Autodesk Fusion 360 part; units mm, degrees
(part 3 of 3)
sketch "b left circles" plane through (0, 0, 0) normal (0, 0, 1) x (1, 0, 0) in component "b left component"
  line L0 (104.02, 122.01) -> (154.02, 122.01)
  line L1 (154.02, 122.01) -> (154.02, 242.01)
  line L2 (154.02, 242.01) -> (104.02, 242.01)
  line L3 (104.02, 242.01) -> (104.02, 122.01)
  circle A0 centre (114.7106, 124.3744) radius 1.005
  circle A1 centre (123.3294, 124.3744) radius 1.005
  circle A2 centre (134.7106, 124.3744) radius 1.005
  circle A3 centre (143.3294, 124.3744) radius 1.005
  circle A4 centre (151.6556, 136.3194) radius 1.005
  circle A5 centre (151.6556, 147.7006) radius 1.005
  circle A6 centre (151.6556, 156.3194) radius 1.005
  circle A7 centre (151.6556, 167.7006) radius 1.005
  circle A8 centre (151.6556, 176.3194) radius 1.005
  circle A9 centre (151.6556, 187.7006) radius 1.005
  circle A10 centre (151.6556, 196.3194) radius 1.005
  circle A11 centre (151.6556, 207.7006) radius 1.005
  circle A12 centre (151.6556, 216.3194) radius 1.005
  circle A13 centre (151.6556, 227.7006) radius 1.005
  circle A14 centre (114.7106, 239.6456) radius 1.005
  circle A15 centre (123.3294, 239.6456) radius 1.005
  circle A16 centre (134.7106, 239.6456) radius 1.005
  circle A17 centre (143.3294, 239.6456) radius 1.005
  circle A18 centre (106.3844, 136.3194) radius 1.005
  circle A19 centre (106.3844, 147.7006) radius 1.005
  circle A20 centre (106.3844, 156.3194) radius 1.005
  circle A21 centre (106.3844, 167.7006) radius 1.005
  circle A22 centre (106.3844, 176.3194) radius 1.005
  circle A23 centre (106.3844, 187.7006) radius 1.005
  circle A24 centre (106.3844, 196.3194) radius 1.005
  circle A25 centre (106.3844, 207.7006) radius 1.005
  circle A26 centre (106.3844, 216.3194) radius 1.005
  circle A27 centre (106.3844, 227.7006) radius 1.005
  dimension "d1976" = 2.01
  dimension "d1977" = 2.01
  dimension "d1978" = 2.01
  dimension "d1979" = 2.01
  dimension "d2001" = 2.01
  dimension "d2002" = 2.01
  dimension "d2003" = 2.01
  dimension "d2004" = 2.01
  dimension "d2005" = 2.01
  dimension "d2006" = 2.01
  dimension "d2007" = 2.01
  dimension "d2008" = 2.01
  dimension "d2009" = 2.01
  dimension "d2010" = 2.01
  dimension "d2020" = 2.01
  dimension "d2021" = 2.01
  dimension "d2022" = 2.01
  dimension "d2023" = 2.01
  dimension "d2045" = 2.01
  dimension "d2046" = 2.01
  dimension "d2047" = 2.01
  dimension "d2048" = 2.01
  dimension "d2049" = 2.01
  dimension "d2050" = 2.01
  dimension "d2051" = 2.01
  dimension "d2052" = 2.01
  dimension "d2053" = 2.01
  dimension "d2054" = 2.01
  measures "d1976" diameter of A0
  measures "d1977" diameter of A1
  measures "d1978" diameter of A2
  measures "d1979" diameter of A3
  measures "d2001" diameter of A4
  measures "d2002" diameter of A5
  measures "d2003" diameter of A6
  measures "d2004" diameter of A7
  measures "d2005" diameter of A8
  measures "d2006" diameter of A9
  measures "d2007" diameter of A10
  measures "d2008" diameter of A11
  measures "d2009" diameter of A12
  measures "d2010" diameter of A13
  measures "d2020" diameter of A14
  measures "d2021" diameter of A15
  measures "d2022" diameter of A16
  measures "d2023" diameter of A17
  measures "d2045" diameter of A18
  measures "d2046" diameter of A19
  measures "d2047" diameter of A20
  measures "d2048" diameter of A21
  measures "d2049" diameter of A22
  measures "d2050" diameter of A23
  measures "d2051" diameter of A24
  measures "d2052" diameter of A25
  measures "d2053" diameter of A26
  measures "d2054" diameter of A27
extrude "b left lines body extrude" add sketch "b left lines" along normal blind 3.175 separate body makes body 10 in component "b left component"
extrude "b left circles extrude" add sketch "b left circles" along normal blind 3.175 separate body makes body 11 in component "b left component"
combine "b left lines final combine feature" operation intersect target body 10 tool bodies 11 in component "b left component"
sketch "b right lines" plane through (0, 0, 0) normal (0, 0, 1) x (1, 0, 0) in component "b right component"
  line L0 (159.205, 122.01) -> (166.13, 122.01)
  line L1 (166.13, 122.01) -> (166.13, 125.185)
  line L2 (166.13, 125.185) -> (175.93, 125.185)
  line L3 (175.93, 125.185) -> (175.93, 122.01)
  line L4 (175.93, 122.01) -> (186.13, 122.01)
  line L5 (186.13, 122.01) -> (186.13, 125.185)
  line L6 (186.13, 125.185) -> (195.93, 125.185)
  line L7 (195.93, 125.185) -> (195.93, 122.01)
  line L8 (195.93, 122.01) -> (202.855, 122.01)
  line L9 (202.855, 122.01) -> (202.855, 136.91)
  line L10 (202.855, 136.91) -> (206.03, 136.91)
  line L11 (206.03, 136.91) -> (206.03, 147.11)
  line L12 (206.03, 147.11) -> (202.855, 147.11)
  line L13 (202.855, 147.11) -> (202.855, 156.91)
  line L14 (202.855, 156.91) -> (206.03, 156.91)
  line L15 (206.03, 156.91) -> (206.03, 167.11)
  line L16 (206.03, 167.11) -> (202.855, 167.11)
  line L17 (202.855, 167.11) -> (202.855, 176.91)
  line L18 (202.855, 176.91) -> (206.03, 176.91)
  line L19 (206.03, 176.91) -> (206.03, 187.11)
  line L20 (206.03, 187.11) -> (202.855, 187.11)
  line L21 (202.855, 187.11) -> (202.855, 196.91)
  line L22 (202.855, 196.91) -> (206.03, 196.91)
  line L23 (206.03, 196.91) -> (206.03, 207.11)
  line L24 (206.03, 207.11) -> (202.855, 207.11)
  line L25 (202.855, 207.11) -> (202.855, 216.91)
  line L26 (202.855, 216.91) -> (206.03, 216.91)
  line L27 (206.03, 216.91) -> (206.03, 227.11)
  line L28 (206.03, 227.11) -> (202.855, 227.11)
  line L29 (202.855, 227.11) -> (202.855, 242.01)
  line L30 (159.205, 242.01) -> (166.13, 242.01)
  line L31 (166.13, 242.01) -> (166.13, 238.835)
  line L32 (166.13, 238.835) -> (175.93, 238.835)
  line L33 (175.93, 238.835) -> (175.93, 242.01)
  line L34 (175.93, 242.01) -> (186.13, 242.01)
  line L35 (186.13, 242.01) -> (186.13, 238.835)
  line L36 (186.13, 238.835) -> (195.93, 238.835)
  line L37 (195.93, 238.835) -> (195.93, 242.01)
  line L38 (195.93, 242.01) -> (202.855, 242.01)
  line L39 (159.205, 122.01) -> (159.205, 136.91)
  line L40 (159.205, 136.91) -> (156.03, 136.91)
  line L41 (156.03, 136.91) -> (156.03, 147.11)
  line L42 (156.03, 147.11) -> (159.205, 147.11)
  line L43 (159.205, 147.11) -> (159.205, 156.91)
  line L44 (159.205, 156.91) -> (156.03, 156.91)
  line L45 (156.03, 156.91) -> (156.03, 167.11)
  line L46 (156.03, 167.11) -> (159.205, 167.11)
  line L47 (159.205, 167.11) -> (159.205, 176.91)
  line L48 (159.205, 176.91) -> (156.03, 176.91)
  line L49 (156.03, 176.91) -> (156.03, 187.11)
  line L50 (156.03, 187.11) -> (159.205, 187.11)
  line L51 (159.205, 187.11) -> (159.205, 196.91)
  line L52 (159.205, 196.91) -> (156.03, 196.91)
  line L53 (156.03, 196.91) -> (156.03, 207.11)
  line L54 (156.03, 207.11) -> (159.205, 207.11)
  line L55 (159.205, 207.11) -> (159.205, 216.91)
  line L56 (159.205, 216.91) -> (156.03, 216.91)
  line L57 (156.03, 216.91) -> (156.03, 227.11)
  line L58 (156.03, 227.11) -> (159.205, 227.11)
  line L59 (159.205, 227.11) -> (159.205, 242.01)
  dimension "d2059" = 6.925
  dimension "d2060" = 3.175
  dimension "d2061" = 9.8
  dimension "d2062" = 3.175
  dimension "d2063" = 10.2
  dimension "d2064" = 3.175
  dimension "d2065" = 9.8
  dimension "d2066" = 3.175
  dimension "d2067" = 6.925
  dimension "d2072" = 14.9
  dimension "d2073" = 3.175
  dimension "d2074" = 10.2
  dimension "d2075" = 3.175
  dimension "d2076" = 9.8
  dimension "d2077" = 3.175
  dimension "d2078" = 10.2
  dimension "d2079" = 3.175
  dimension "d2080" = 9.8
  dimension "d2081" = 3.175
  dimension "d2082" = 10.2
  dimension "d2083" = 3.175
  dimension "d2084" = 9.8
  dimension "d2085" = 3.175
  dimension "d2086" = 10.2
  dimension "d2087" = 3.175
  dimension "d2088" = 9.8
  dimension "d2089" = 3.175
  dimension "d2090" = 10.2
  dimension "d2091" = 3.175
  dimension "d2092" = 14.9
  dimension "d2103" = 6.925
  dimension "d2104" = 3.175
  dimension "d2105" = 9.8
  dimension "d2106" = 3.175
  dimension "d2107" = 10.2
  dimension "d2108" = 3.175
  dimension "d2109" = 9.8
  dimension "d2110" = 3.175
  dimension "d2111" = 6.925
  dimension "d2116" = 14.9
  dimension "d2117" = 3.175
  dimension "d2118" = 10.2
  dimension "d2119" = 3.175
  dimension "d2120" = 9.8
  dimension "d2121" = 3.175
  dimension "d2122" = 10.2
  dimension "d2123" = 3.175
  dimension "d2124" = 9.8
  dimension "d2125" = 3.175
  dimension "d2126" = 10.2
  dimension "d2127" = 3.175
  dimension "d2128" = 9.8
  dimension "d2129" = 3.175
  dimension "d2130" = 10.2
  dimension "d2131" = 3.175
  dimension "d2132" = 9.8
  dimension "d2133" = 3.175
  dimension "d2134" = 10.2
  dimension "d2135" = 3.175
  dimension "d2136" = 14.9
  constraint horizontal L0
  constraint vertical L1
  constraint horizontal L2
  constraint vertical L3
  constraint horizontal L4
  constraint vertical L5
  constraint horizontal L6
  constraint vertical L7
  constraint horizontal L8
  constraint vertical L9
  constraint horizontal L10
  constraint vertical L11
  constraint horizontal L12
  constraint vertical L13
  constraint horizontal L14
  constraint vertical L15
  constraint horizontal L16
  constraint vertical L17
  constraint horizontal L18
  constraint vertical L19
  constraint horizontal L20
  constraint vertical L21
  constraint horizontal L22
  constraint vertical L23
  constraint horizontal L24
  constraint vertical L25
  constraint horizontal L26
  constraint vertical L27
  constraint horizontal L28
  constraint vertical L29
  constraint horizontal L30
  constraint vertical L31
  constraint horizontal L32
  constraint vertical L33
  constraint horizontal L34
  constraint vertical L35
  constraint horizontal L36
  constraint vertical L37
  constraint horizontal L38
  constraint vertical L39
  constraint horizontal L40
  constraint vertical L41
  constraint horizontal L42
  constraint vertical L43
  constraint horizontal L44
  constraint vertical L45
  constraint horizontal L46
  constraint vertical L47
  constraint horizontal L48
  constraint vertical L49
  constraint horizontal L50
  constraint vertical L51
  constraint horizontal L52
  constraint vertical L53
  constraint horizontal L54
  constraint vertical L55
  constraint horizontal L56
  constraint vertical L57
  constraint horizontal L58
  constraint vertical L59
  measures "d2059" distance of L0.start L0.end
  measures "d2060" distance of L0.end L1.end
  measures "d2061" distance of L1.end L2.end
  measures "d2062" distance of L2.end L3.end
  measures "d2063" distance of L3.end L4.end
  measures "d2064" distance of L4.end L5.end
  measures "d2065" distance of L5.end L6.end
  measures "d2066" distance of L6.end L7.end
  measures "d2067" distance of L7.end L8.end
  measures "d2072" distance of L8.end L9.end
  measures "d2073" distance of L9.end L10.end
  measures "d2074" distance of L10.end L11.end
  measures "d2075" distance of L11.end L12.end
  measures "d2076" distance of L12.end L13.end
  measures "d2077" distance of L13.end L14.end
  measures "d2078" distance of L14.end L15.end
  measures "d2079" distance of L15.end L16.end
  measures "d2080" distance of L16.end L17.end
  measures "d2081" distance of L17.end L18.end
  measures "d2082" distance of L18.end L19.end
  measures "d2083" distance of L19.end L20.end
  measures "d2084" distance of L20.end L21.end
  measures "d2085" distance of L21.end L22.end
  measures "d2086" distance of L22.end L23.end
  measures "d2087" distance of L23.end L24.end
  measures "d2088" distance of L24.end L25.end
  measures "d2089" distance of L25.end L26.end
  measures "d2090" distance of L26.end L27.end
  measures "d2091" distance of L27.end L28.end
  measures "d2092" distance of L28.end L29.end
  measures "d2103" distance of L30.start L30.end
  measures "d2104" distance of L30.end L31.end
  measures "d2105" distance of L31.end L32.end
  measures "d2106" distance of L32.end L33.end
  measures "d2107" distance of L33.end L34.end
  measures "d2108" distance of L34.end L35.end
  measures "d2109" distance of L35.end L36.end
  measures "d2110" distance of L36.end L37.end
  measures "d2111" distance of L29.end L37.end
  measures "d2116" distance of L0.start L39.end
  measures "d2117" distance of L39.end L40.end
  measures "d2118" distance of L40.end L41.end
  measures "d2119" distance of L41.end L42.end
  measures "d2120" distance of L42.end L43.end
  measures "d2121" distance of L43.end L44.end
  measures "d2122" distance of L44.end L45.end
  measures "d2123" distance of L45.end L46.end
  measures "d2124" distance of L46.end L47.end
  measures "d2125" distance of L47.end L48.end
  measures "d2126" distance of L48.end L49.end
  measures "d2127" distance of L49.end L50.end
  measures "d2128" distance of L50.end L51.end
  measures "d2129" distance of L51.end L52.end
  measures "d2130" distance of L52.end L53.end
  measures "d2131" distance of L53.end L54.end
  measures "d2132" distance of L54.end L55.end
  measures "d2133" distance of L55.end L56.end
  measures "d2134" distance of L56.end L57.end
  measures "d2135" distance of L57.end L58.end
  measures "d2136" distance of L30.start L58.end
sketch "b right circles" plane through (0, 0, 0) normal (0, 0, 1) x (1, 0, 0) in component "b right component"
  line L0 (156.03, 122.01) -> (206.03, 122.01)
  line L1 (206.03, 122.01) -> (206.03, 242.01)
  line L2 (206.03, 242.01) -> (156.03, 242.01)
  line L3 (156.03, 242.01) -> (156.03, 122.01)
  circle A0 centre (166.7206, 124.3744) radius 1.005
  circle A1 centre (175.3394, 124.3744) radius 1.005
  circle A2 centre (186.7206, 124.3744) radius 1.005
  circle A3 centre (195.3394, 124.3744) radius 1.005
  circle A4 centre (203.6656, 136.3194) radius 1.005
  circle A5 centre (203.6656, 147.7006) radius 1.005
  circle A6 centre (203.6656, 156.3194) radius 1.005
  circle A7 centre (203.6656, 167.7006) radius 1.005
  circle A8 centre (203.6656, 176.3194) radius 1.005
  circle A9 centre (203.6656, 187.7006) radius 1.005
  circle A10 centre (203.6656, 196.3194) radius 1.005
  circle A11 centre (203.6656, 207.7006) radius 1.005
  circle A12 centre (203.6656, 216.3194) radius 1.005
  circle A13 centre (203.6656, 227.7006) radius 1.005
  circle A14 centre (166.7206, 239.6456) radius 1.005
  circle A15 centre (175.3394, 239.6456) radius 1.005
  circle A16 centre (186.7206, 239.6456) radius 1.005
  circle A17 centre (195.3394, 239.6456) radius 1.005
  circle A18 centre (158.3944, 136.3194) radius 1.005
  circle A19 centre (158.3944, 147.7006) radius 1.005
  circle A20 centre (158.3944, 156.3194) radius 1.005
  circle A21 centre (158.3944, 167.7006) radius 1.005
  circle A22 centre (158.3944, 176.3194) radius 1.005
  circle A23 centre (158.3944, 187.7006) radius 1.005
  circle A24 centre (158.3944, 196.3194) radius 1.005
  circle A25 centre (158.3944, 207.7006) radius 1.005
  circle A26 centre (158.3944, 216.3194) radius 1.005
  circle A27 centre (158.3944, 227.7006) radius 1.005
  dimension "d2068" = 2.01
  dimension "d2069" = 2.01
  dimension "d2070" = 2.01
  dimension "d2071" = 2.01
  dimension "d2093" = 2.01
  dimension "d2094" = 2.01
  dimension "d2095" = 2.01
  dimension "d2096" = 2.01
  dimension "d2097" = 2.01
  dimension "d2098" = 2.01
  dimension "d2099" = 2.01
  dimension "d2100" = 2.01
  dimension "d2101" = 2.01
  dimension "d2102" = 2.01
  dimension "d2112" = 2.01
  dimension "d2113" = 2.01
  dimension "d2114" = 2.01
  dimension "d2115" = 2.01
  dimension "d2137" = 2.01
  dimension "d2138" = 2.01
  dimension "d2139" = 2.01
  dimension "d2140" = 2.01
  dimension "d2141" = 2.01
  dimension "d2142" = 2.01
  dimension "d2143" = 2.01
  dimension "d2144" = 2.01
  dimension "d2145" = 2.01
  dimension "d2146" = 2.01
  measures "d2068" diameter of A0
  measures "d2069" diameter of A1
  measures "d2070" diameter of A2
  measures "d2071" diameter of A3
  measures "d2093" diameter of A4
  measures "d2094" diameter of A5
  measures "d2095" diameter of A6
  measures "d2096" diameter of A7
  measures "d2097" diameter of A8
  measures "d2098" diameter of A9
  measures "d2099" diameter of A10
  measures "d2100" diameter of A11
  measures "d2101" diameter of A12
  measures "d2102" diameter of A13
  measures "d2112" diameter of A14
  measures "d2113" diameter of A15
  measures "d2114" diameter of A16
  measures "d2115" diameter of A17
  measures "d2137" diameter of A18
  measures "d2138" diameter of A19
  measures "d2139" diameter of A20
  measures "d2140" diameter of A21
  measures "d2141" diameter of A22
  measures "d2142" diameter of A23
  measures "d2143" diameter of A24
  measures "d2144" diameter of A25
  measures "d2145" diameter of A26
  measures "d2146" diameter of A27
extrude "b right lines body extrude" add sketch "b right lines" along normal blind 3.175 separate body makes body 12 in component "b right component"
extrude "b right circles extrude" add sketch "b right circles" along normal blind 3.175 separate body makes body 13 in component "b right component"
combine "b right lines final combine feature" operation intersect target body 12 tool bodies 13 in component "b right component"
component "b top component" placed x (1, 0, 0) y (0, 1, 0) z (0, 0, 1) at (0, 0, 0)
component "b bottom component" placed x (1, 0, 0) y (0, 1, 0) z (0, 0, 1) at (0, 0, 0)
component "b front component" placed x (1, 0, 0) y (0, 1, 0) z (0, 0, 1) at (0, 0, 0)
component "b back component" placed x (1, 0, 0) y (0, 1, 0) z (0, 0, 1) at (0, 0, 0)
component "b left component" placed x (1, 0, 0) y (0, 1, 0) z (0, 0, 1) at (0, 0, 0)
component "b right component" placed x (1, 0, 0) y (0, 1, 0) z (0, 0, 1) at (0, 0, 0)
equation "toolDiameter = 2.01 mm"
equation "d272 = screwHoleSize"
equation "d282 = pcbMountHoles"
equation "d289 = pcbMountHoles"
equation "screwHoleSize = 3.176 mm"
equation "d366 = pcbMountHoles"
equation "pcbMountHoles = 2 mm"
equation "d368 = pcbMountHoles"
equation "d369 = pcbMountHoles"
equation "d370 = pcbMountHoles"
equation "d391 = toolDiameter"
equation "d402 = toolDiameter"
equation "Version_info = 0 mm" comment "1.0.0 LENGTH 150 DEPTH 120 HEIGHT 50 THICKNESS 3.175 TOOL_DIAMETER 2.01 TOOTH_WIDTH 10 KERF -0.1 DELTA_FROM_BOTTOM -0.1 STOCK_X_DIMENSION 304.8 STOCK_Y_DIMENSION 609.6 COMPONENT   REPEATS_L_TMP -1 CREATE_COMPONENTS False CREATE_BODIES 1 CREATE_EMPTY_CONTENTS False CREATE_CONSTRAINTS True CLEAR_PREVIOUSLY_GENERATED_ITEMS True JUST_CLEAR_PREVIOUSLY_GENERATED_ITEMS False CREATE_MANUFACTURING False CREATE_LAYOUT True DEBUG_JUST_ONE_PART True DEBUG True"
equation "Length = 150.0 mm" comment "Length (mm)"
equation "Depth = 120.0 mm" comment "Depth (mm)"
equation "Height = 50.0 mm" comment "Height (mm)"
equation "Thickness = 3.175 mm" comment "Thickness (mm)"
equation "Tool_diameter = 2.01 mm" comment "Tool Diameter (mm)"
equation "Tooth_width = 10.0 mm" comment "Target Tooth Width (mm)"
equation "Kerf = -0.1 mm" comment "Kerf (mm)- can be negative"
equation "Delta_from_bottom = -0.1 mm" comment "Additional fine adjustment of bone centers from bottom of holes(mm)- positive makes smaller bottom indents"
equation "Stock_x_dimension = 304.8 mm" comment "Stock X Dimension"
equation "Stock_y_dimension = 609.6 mm" comment "Stock Y Dimension"
equation "Repeats_l_tmp = -1.0 mm" comment "temp hidden"
equation "d1432 = Thickness"
equation "d1434 = Thickness"
equation "d1436 = Thickness"
equation "d1438 = Thickness"
equation "d1440 = Thickness"
equation "d1442 = Thickness"
equation "d1444 = Thickness"
equation "d1446 = Thickness"
equation "d1448 = Thickness"
equation "d1450 = Thickness"
equation "d1452 = Thickness"
equation "d1454 = Thickness"
equation "d1456 = Thickness"
equation "d1458 = Thickness"
equation "d1460 = Tool_diameter"
equation "d1461 = Tool_diameter"
equation "d1462 = Tool_diameter"
equation "d1463 = Tool_diameter"
equation "d1464 = Tool_diameter"
equation "d1465 = Tool_diameter"
equation "d1466 = Tool_diameter"
equation "d1467 = Tool_diameter"
equation "d1468 = Tool_diameter"
equation "d1469 = Tool_diameter"
equation "d1470 = Tool_diameter"
equation "d1471 = Tool_diameter"
equation "d1472 = Tool_diameter"
equation "d1473 = Tool_diameter"
equation "d1475 = Thickness"
equation "d1477 = Thickness"
equation "d1479 = Thickness"
equation "d1481 = Thickness"
equation "d1483 = Thickness"
equation "d1485 = Thickness"
equation "d1487 = Thickness"
equation "d1489 = Thickness"
equation "d1491 = Thickness"
equation "d1493 = Thickness"
equation "d1495 = Tool_diameter"
equation "d1496 = Tool_diameter"
equation "d1497 = Tool_diameter"
equation "d1498 = Tool_diameter"
equation "d1499 = Tool_diameter"
equation "d1500 = Tool_diameter"
equation "d1501 = Tool_diameter"
equation "d1502 = Tool_diameter"
equation "d1503 = Tool_diameter"
equation "d1504 = Tool_diameter"
equation "d1506 = Thickness"
equation "d1508 = Thickness"
equation "d1510 = Thickness"
equation "d1512 = Thickness"
equation "d1514 = Thickness"
equation "d1516 = Thickness"
equation "d1518 = Thickness"
equation "d1520 = Thickness"
equation "d1522 = Thickness"
equation "d1524 = Thickness"
equation "d1526 = Thickness"
equation "d1528 = Thickness"
equation "d1530 = Thickness"
equation "d1532 = Thickness"
equation "d1534 = Tool_diameter"
equation "d1535 = Tool_diameter"
equation "d1536 = Tool_diameter"
equation "d1537 = Tool_diameter"
equation "d1538 = Tool_diameter"
equation "d1539 = Tool_diameter"
equation "d1540 = Tool_diameter"
equation "d1541 = Tool_diameter"
equation "d1542 = Tool_diameter"
equation "d1543 = Tool_diameter"
equation "d1544 = Tool_diameter"
equation "d1545 = Tool_diameter"
equation "d1546 = Tool_diameter"
equation "d1547 = Tool_diameter"
equation "d1549 = Thickness"
equation "d1551 = Thickness"
equation "d1553 = Thickness"
equation "d1555 = Thickness"
equation "d1557 = Thickness"
equation "d1559 = Thickness"
equation "d1561 = Thickness"
equation "d1563 = Thickness"
equation "d1565 = Thickness"
equation "d1567 = Thickness"
equation "d1569 = Tool_diameter"
equation "d1570 = Tool_diameter"
equation "d1571 = Tool_diameter"
equation "d1572 = Tool_diameter"
equation "d1573 = Tool_diameter"
equation "d1574 = Tool_diameter"
equation "d1575 = Tool_diameter"
equation "d1576 = Tool_diameter"
equation "d1577 = Tool_diameter"
equation "d1578 = Tool_diameter"
equation "d1584 = Thickness"
equation "d1586 = Thickness"
equation "d1588 = Thickness"
equation "d1590 = Thickness"
equation "d1592 = Thickness"
equation "d1594 = Thickness"
equation "d1596 = Thickness"
equation "d1598 = Thickness"
equation "d1600 = Thickness"
equation "d1602 = Thickness"
equation "d1604 = Thickness"
equation "d1606 = Thickness"
equation "d1608 = Thickness"
equation "d1610 = Thickness"
equation "d1612 = Tool_diameter"
equation "d1613 = Tool_diameter"
equation "d1614 = Tool_diameter"
equation "d1615 = Tool_diameter"
equation "d1616 = Tool_diameter"
equation "d1617 = Tool_diameter"
equation "d1618 = Tool_diameter"
equation "d1619 = Tool_diameter"
equation "d1620 = Tool_diameter"
equation "d1621 = Tool_diameter"
equation "d1622 = Tool_diameter"
equation "d1623 = Tool_diameter"
equation "d1624 = Tool_diameter"
equation "d1625 = Tool_diameter"
equation "d1627 = Thickness"
equation "d1629 = Thickness"
equation "d1631 = Thickness"
equation "d1633 = Thickness"
equation "d1635 = Thickness"
equation "d1637 = Thickness"
equation "d1639 = Thickness"
equation "d1641 = Thickness"
equation "d1643 = Thickness"
equation "d1645 = Thickness"
equation "d1647 = Tool_diameter"
equation "d1648 = Tool_diameter"
equation "d1649 = Tool_diameter"
equation "d1650 = Tool_diameter"
equation "d1651 = Tool_diameter"
equation "d1652 = Tool_diameter"
equation "d1653 = Tool_diameter"
equation "d1654 = Tool_diameter"
equation "d1655 = Tool_diameter"
equation "d1656 = Tool_diameter"
equation "d1658 = Thickness"
equation "d1660 = Thickness"
equation "d1662 = Thickness"
equation "d1664 = Thickness"
equation "d1666 = Thickness"
equation "d1668 = Thickness"
equation "d1670 = Thickness"
equation "d1672 = Thickness"
equation "d1674 = Thickness"
equation "d1676 = Thickness"
equation "d1678 = Thickness"
equation "d1680 = Thickness"
equation "d1682 = Thickness"
equation "d1684 = Thickness"
equation "d1686 = Tool_diameter"
equation "d1687 = Tool_diameter"
equation "d1688 = Tool_diameter"
equation "d1689 = Tool_diameter"
equation "d1690 = Tool_diameter"
equation "d1691 = Tool_diameter"
equation "d1692 = Tool_diameter"
equation "d1693 = Tool_diameter"
equation "d1694 = Tool_diameter"
equation "d1695 = Tool_diameter"
equation "d1696 = Tool_diameter"
equation "d1697 = Tool_diameter"
equation "d1698 = Tool_diameter"
equation "d1699 = Tool_diameter"
equation "d1701 = Thickness"
equation "d1703 = Thickness"
equation "d1705 = Thickness"
equation "d1707 = Thickness"
equation "d1709 = Thickness"
equation "d1711 = Thickness"
equation "d1713 = Thickness"
equation "d1715 = Thickness"
equation "d1717 = Thickness"
equation "d1719 = Thickness"
equation "d1721 = Tool_diameter"
equation "d1722 = Tool_diameter"
equation "d1723 = Tool_diameter"
equation "d1724 = Tool_diameter"
equation "d1725 = Tool_diameter"
equation "d1726 = Tool_diameter"
equation "d1727 = Tool_diameter"
equation "d1728 = Tool_diameter"
equation "d1729 = Tool_diameter"
equation "d1730 = Tool_diameter"
equation "d1736 = Thickness"
equation "d1738 = Thickness"
equation "d1740 = Thickness"
equation "d1742 = Thickness"
equation "d1744 = Tool_diameter"
equation "d1745 = Tool_diameter"
equation "d1746 = Tool_diameter"
equation "d1747 = Tool_diameter"
equation "d1749 = Thickness"
equation "d1751 = Thickness"
equation "d1753 = Thickness"
equation "d1755 = Thickness"
equation "d1757 = Thickness"
equation "d1759 = Thickness"
equation "d1761 = Thickness"
equation "d1763 = Thickness"
equation "d1765 = Thickness"
equation "d1767 = Thickness"
equation "d1769 = Thickness"
equation "d1771 = Thickness"
equation "d1773 = Thickness"
equation "d1775 = Thickness"
equation "d1777 = Tool_diameter"
equation "d1778 = Tool_diameter"
equation "d1779 = Tool_diameter"
equation "d1780 = Tool_diameter"
equation "d1781 = Tool_diameter"
equation "d1782 = Tool_diameter"
equation "d1783 = Tool_diameter"
equation "d1784 = Tool_diameter"
equation "d1785 = Tool_diameter"
equation "d1786 = Tool_diameter"
equation "d1787 = Tool_diameter"
equation "d1788 = Tool_diameter"
equation "d1789 = Tool_diameter"
equation "d1790 = Tool_diameter"
equation "d1792 = Thickness"
equation "d1794 = Thickness"
equation "d1796 = Thickness"
equation "d1798 = Thickness"
equation "d1800 = Tool_diameter"
equation "d1801 = Tool_diameter"
equation "d1802 = Tool_diameter"
equation "d1803 = Tool_diameter"
equation "d1805 = Thickness"
equation "d1807 = Thickness"
equation "d1809 = Thickness"
equation "d1811 = Thickness"
equation "d1813 = Thickness"
equation "d1815 = Thickness"
equation "d1817 = Thickness"
equation "d1819 = Thickness"
equation "d1821 = Thickness"
equation "d1823 = Thickness"
equation "d1825 = Thickness"
equation "d1827 = Thickness"
equation "d1829 = Thickness"
equation "d1831 = Thickness"
equation "d1833 = Tool_diameter"
equation "d1834 = Tool_diameter"
equation "d1835 = Tool_diameter"
equation "d1836 = Tool_diameter"
equation "d1837 = Tool_diameter"
equation "d1838 = Tool_diameter"
equation "d1839 = Tool_diameter"
equation "d1840 = Tool_diameter"
equation "d1841 = Tool_diameter"
equation "d1842 = Tool_diameter"
equation "d1843 = Tool_diameter"
equation "d1844 = Tool_diameter"
equation "d1845 = Tool_diameter"
equation "d1846 = Tool_diameter"
equation "d1852 = Thickness"
equation "d1854 = Thickness"
equation "d1856 = Thickness"
equation "d1858 = Thickness"
equation "d1860 = Tool_diameter"
equation "d1861 = Tool_diameter"
equation "d1862 = Tool_diameter"
equation "d1863 = Tool_diameter"
equation "d1865 = Thickness"
equation "d1867 = Thickness"
equation "d1869 = Thickness"
equation "d1871 = Thickness"
equation "d1873 = Thickness"
equation "d1875 = Thickness"
equation "d1877 = Thickness"
equation "d1879 = Thickness"
equation "d1881 = Thickness"
equation "d1883 = Thickness"
equation "d1885 = Thickness"
equation "d1887 = Thickness"
equation "d1889 = Thickness"
equation "d1891 = Thickness"
equation "d1893 = Tool_diameter"
equation "d1894 = Tool_diameter"
equation "d1895 = Tool_diameter"
equation "d1896 = Tool_diameter"
equation "d1897 = Tool_diameter"
equation "d1898 = Tool_diameter"
equation "d1899 = Tool_diameter"
equation "d1900 = Tool_diameter"
equation "d1901 = Tool_diameter"
equation "d1902 = Tool_diameter"
equation "d1903 = Tool_diameter"
equation "d1904 = Tool_diameter"
equation "d1905 = Tool_diameter"
equation "d1906 = Tool_diameter"
equation "d1908 = Thickness"
equation "d1910 = Thickness"
equation "d1912 = Thickness"
equation "d1914 = Thickness"
equation "d1916 = Tool_diameter"
equation "d1917 = Tool_diameter"
equation "d1918 = Tool_diameter"
equation "d1919 = Tool_diameter"
equation "d1921 = Thickness"
equation "d1923 = Thickness"
equation "d1925 = Thickness"
equation "d1927 = Thickness"
equation "d1929 = Thickness"
equation "d1931 = Thickness"
equation "d1933 = Thickness"
equation "d1935 = Thickness"
equation "d1937 = Thickness"
equation "d1939 = Thickness"
equation "d1941 = Thickness"
equation "d1943 = Thickness"
equation "d1945 = Thickness"
equation "d1947 = Thickness"
equation "d1949 = Tool_diameter"
equation "d1950 = Tool_diameter"
equation "d1951 = Tool_diameter"
equation "d1952 = Tool_diameter"
equation "d1953 = Tool_diameter"
equation "d1954 = Tool_diameter"
equation "d1955 = Tool_diameter"
equation "d1956 = Tool_diameter"
equation "d1957 = Tool_diameter"
equation "d1958 = Tool_diameter"
equation "d1959 = Tool_diameter"
equation "d1960 = Tool_diameter"
equation "d1961 = Tool_diameter"
equation "d1962 = Tool_diameter"
equation "d1968 = Thickness"
equation "d1970 = Thickness"
equation "d1972 = Thickness"
equation "d1974 = Thickness"
equation "d1976 = Tool_diameter"
equation "d1977 = Tool_diameter"
equation "d1978 = Tool_diameter"
equation "d1979 = Tool_diameter"
equation "d1981 = Thickness"
equation "d1983 = Thickness"
equation "d1985 = Thickness"
equation "d1987 = Thickness"
equation "d1989 = Thickness"
equation "d1991 = Thickness"
equation "d1993 = Thickness"
equation "d1995 = Thickness"
equation "d1997 = Thickness"
equation "d1999 = Thickness"
equation "d2001 = Tool_diameter"
equation "d2002 = Tool_diameter"
equation "d2003 = Tool_diameter"
equation "d2004 = Tool_diameter"
equation "d2005 = Tool_diameter"
equation "d2006 = Tool_diameter"
equation "d2007 = Tool_diameter"
equation "d2008 = Tool_diameter"
equation "d2009 = Tool_diameter"
equation "d2010 = Tool_diameter"
equation "d2012 = Thickness"
equation "d2014 = Thickness"
equation "d2016 = Thickness"
equation "d2018 = Thickness"
equation "d2020 = Tool_diameter"
equation "d2021 = Tool_diameter"
equation "d2022 = Tool_diameter"
equation "d2023 = Tool_diameter"
equation "d2025 = Thickness"
equation "d2027 = Thickness"
equation "d2029 = Thickness"
equation "d2031 = Thickness"
equation "d2033 = Thickness"
equation "d2035 = Thickness"
equation "d2037 = Thickness"
equation "d2039 = Thickness"
equation "d2041 = Thickness"
equation "d2043 = Thickness"
equation "d2045 = Tool_diameter"
equation "d2046 = Tool_diameter"
equation "d2047 = Tool_diameter"
equation "d2048 = Tool_diameter"
equation "d2049 = Tool_diameter"
equation "d2050 = Tool_diameter"
equation "d2051 = Tool_diameter"
equation "d2052 = Tool_diameter"
equation "d2053 = Tool_diameter"
equation "d2054 = Tool_diameter"
equation "d2060 = Thickness"
equation "d2062 = Thickness"
equation "d2064 = Thickness"
equation "d2066 = Thickness"
equation "d2068 = Tool_diameter"
equation "d2069 = Tool_diameter"
equation "d2070 = Tool_diameter"
equation "d2071 = Tool_diameter"
equation "d2073 = Thickness"
equation "d2075 = Thickness"
equation "d2077 = Thickness"
equation "d2079 = Thickness"
equation "d2081 = Thickness"
equation "d2083 = Thickness"
equation "d2085 = Thickness"
equation "d2087 = Thickness"
equation "d2089 = Thickness"
equation "d2091 = Thickness"
equation "d2093 = Tool_diameter"
equation "d2094 = Tool_diameter"
equation "d2095 = Tool_diameter"
equation "d2096 = Tool_diameter"
equation "d2097 = Tool_diameter"
equation "d2098 = Tool_diameter"
equation "d2099 = Tool_diameter"
equation "d2100 = Tool_diameter"
equation "d2101 = Tool_diameter"
equation "d2102 = Tool_diameter"
equation "d2104 = Thickness"
equation "d2106 = Thickness"
equation "d2108 = Thickness"
equation "d2110 = Thickness"
equation "d2112 = Tool_diameter"
equation "d2113 = Tool_diameter"
equation "d2114 = Tool_diameter"
equation "d2115 = Tool_diameter"
equation "d2117 = Thickness"
equation "d2119 = Thickness"
equation "d2121 = Thickness"
equation "d2123 = Thickness"
equation "d2125 = Thickness"
equation "d2127 = Thickness"
equation "d2129 = Thickness"
equation "d2131 = Thickness"
equation "d2133 = Thickness"
equation "d2135 = Thickness"
equation "d2137 = Tool_diameter"
equation "d2138 = Tool_diameter"
equation "d2139 = Tool_diameter"
equation "d2140 = Tool_diameter"
equation "d2141 = Tool_diameter"
equation "d2142 = Tool_diameter"
equation "d2143 = Tool_diameter"
equation "d2144 = Tool_diameter"
equation "d2145 = Tool_diameter"
equation "d2146 = Tool_diameter"
named bodies: "b  stock body", "b top  body", "b top circles cheese body", "b bottom  body", "b bottom circles cheese body", "b front  body", "b front circles cheese body", "b back  body", "b back circles cheese body", "b left  body", "b left circles cheese body", "b right  body", "b right circles cheese body"
